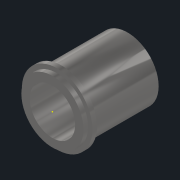
# Autodesk Inventor part: Nut
Saved by Autodesk Inventor 2021 (Build 250183000, 183)
## iProperties
Created: 2020-10-12
Part Number: Nut
Material: Stainless Steel AISI 302
Document SubType Name: Modeling
Designer: Eugene Tang
Mass: 1049.69 g
Surface Area: 340.538 cm^2
Volume: 131.212 cm^3
Density: 8 g/cm^3
Appearance: Semi-Polished
Author: Eugene Tang
Autodesk Inventor part; units mm, degrees
ref_plane "YZ Plane" through (0, 0, 0) normal (1, 0, 0) x (0, 1, 0)
ref_plane "XZ Plane" through (0, 0, 0) normal (0, 1, 0) x (-1, 0, 0)
ref_plane "XY Plane" through (0, 0, 0) normal (0, 0, 1) x (1, 0, 0)
sketch "Sketch1" plane through (0, 0, 0) normal (0, 0, 1) x (1, 0, 0)
  circle A0 centre (0, 0) radius 24.223
  circle A1 centre (0, 0) radius 33
  circle A2 centre (0, 0) radius 18 projected
  dimension "d0" = 6.223
  dimension "d2" = 66
  constraints: 2 centre point, 2 coincident
  measures "d0" radial gap between concentric circles of A0 A2
  measures "d2" diameter of A1
extrude "Nut Ext" add sketch "Sketch1" against normal blind 80 contours A1
ref_plane "Flange Plane" through (0, 0, -5) normal (0, 0, 1) x (1, 0, 0)
sketch "Sketch2" plane through (0, 0, -5) normal (0, 0, 1) x (1, 0, 0)
  circle A0 centre (0, 0) radius 33 projected
  circle A1 centre (0, 0) radius 37.5
  dimension "d6" = 75
  constraints: 1 centre point, 1 coincident
  measures "d6" diameter of A1
extrude "Flange Ext" add sketch "Sketch2" against normal blind 5
ref_plane "Main YZ" through (0, 0, -135.1189) normal (0.9974651, -0.0711568, 0) x (-0.0711568, -0.9974651, 0)
equation "\"d0\" = 2 * d25"
equation "\"d3\" = Nut_L"
equation "\"d6\" = Flange_DIA"
equation "\"d7\" = Flange_L"
equation "\"TD\" = 0.01"
equation "\"Ball_DIA\" = 6.35"
equation "\"Screw_DIA\" = 36"
equation "\"Nut_L\" = 80"
equation "\"Nut_OD\" = 66"
equation "\"Flange_OFFSET\" = 5"
equation "\"d5\" = -Flange_OFFSET"
equation "\"Flange_DIA\" = 75"
equation "\"Flange_L\" = 5"
equation "\"d25\" = 3.1115"
